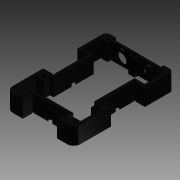
# Autodesk Inventor part: Zwischenebene_Motor2_liegend
Saved by Autodesk Inventor 2015 (Build 190159000, 159)
## iProperties
Created: 2015-03-02
Part Number: Zwischenebene_Motor2_liegend
Material: Generisch
Document SubType Name: Modeling
Designer: TowerSebi
Density: 1 g/cm^3
Appearance: Glatt - schwarz
Author: TowerSebi
Autodesk Inventor part; units mm, degrees
ref_plane "YZ Plane" through (0, 0, 0) normal (1, 0, 0) x (0, 1, 0)
ref_plane "XZ Plane" through (0, 0, 0) normal (0, 1, 0) x (-1, 0, 0)
ref_plane "XY Plane" through (0, 0, 0) normal (0, 0, 1) x (1, 0, 0)
sketch "Skizze1" plane through (0, 0, 0) normal (0, 0, 1) x (1, 0, 0)
  line L0 (0, 0) -> (100, 0)
  line L1 (100, 0) -> (100, 145)
  line L2 (0, 145) -> (0, 0)
  arc A0 (100, 145) -> (0, 145) centre (50, 69.1667) ccw
  dimension "d0" = 145
  dimension "d1" = 100
  constraints: 6 end point, 2 point on circle, 1 centre point, 1 horizontal, 1 parallel, 1 perpendicular
  measures "d0" distance of L2.start L0.start
  measures "d1" distance of L1.end L2.start
extrude "Extrusion1" add sketch "Skizze1" along normal blind 24.5
fillet "Rundung2" radius 10 2 edges at (100, 0, 12.25) (0, 0, 12.25)
fillet "Rundung3" radius 5 2 edges at (100, 145, 12.25) (0, 145, 12.25)
sketch "Skizze3" plane through (0, 0, 0) normal (0, 0, -1) x (-1, 0, 0)
  line L0 (-10, 0) -> (-90, 0) projected
  line L1 (0, 142.2581) -> (0, 10) projected
  circle A0 centre (-90, 10) radius 1.75
  circle A1 centre (-70, 10) radius 1.75
  circle A2 centre (-30, 10) radius 1.75
  circle A3 centre (-10, 10) radius 1.75
  circle A4 centre (-10, 60) radius 1.75
  circle A5 centre (-10, 100) radius 1.75
  circle A6 centre (-10, 140) radius 1.75
  circle A7 centre (-50, 140) radius 1.75
  circle A8 centre (-90, 140) radius 1.75
  circle A9 centre (-90, 100) radius 1.75
  circle A10 centre (-90, 60) radius 1.75
  point P0 (0, 0)
  dimension "d12" = 3.5
  dimension "d13" = 3.5
  dimension "d14" = 3.5
  dimension "d15" = 3.5
  dimension "d16" = 3.5
  dimension "d17" = 3.5
  dimension "d18" = 3.5
  dimension "d19" = 3.5
  dimension "d20" = 3.5
  dimension "d21" = 3.5
  dimension "d22" = 3.5
  dimension "d23" = 140
  dimension "d24" = 140
  dimension "d25" = 140
  dimension "d26" = 100
  dimension "d27" = 100
  dimension "d28" = 60
  dimension "d29" = 60
  dimension "d30" = 10
  dimension "d31" = 10
  dimension "d32" = 10
  dimension "d33" = 10
  dimension "d34" = 90
  dimension "d35" = 70
  dimension "d36" = 30
  dimension "d37" = 10
  dimension "d38" = 90
  dimension "d39" = 10
  dimension "d40" = 90
  dimension "d41" = 10
  dimension "d42" = 90
  dimension "d43" = 50
  dimension "d44" = 10
  constraints: 11 centre point
  measures "d12" diameter of A8
  measures "d13" diameter of A7
  measures "d14" diameter of A6
  measures "d15" diameter of A9
  measures "d16" diameter of A5
  measures "d17" diameter of A10
  measures "d18" diameter of A4
  measures "d19" diameter of A0
  measures "d20" diameter of A1
  measures "d21" diameter of A2
  measures "d22" diameter of A3
  measures "d23" distance from line of L0 A8.centre
  measures "d24" distance from line of L0 A7.centre
  measures "d25" distance from line of L0 A6.centre
  measures "d26" distance from line of L0 A9.centre
  measures "d27" distance from line of L0 A5.centre
  measures "d28" distance from line of L0 A10.centre
  measures "d29" distance from line of L0 A4.centre
  measures "d30" distance from line of L0 A0.centre
  measures "d31" distance from line of A1.centre L0
  measures "d32" distance from line of L0 A2.centre
  measures "d33" distance from line of L0 A3.centre
  measures "d34" distance from line of L1 A0.centre
  measures "d35" distance from line of L1 A1.centre
  measures "d36" distance from line of A2.centre L1
  measures "d37" distance of L1.end A3.centre
  measures "d38" distance from line of L1 A10.centre
  measures "d39" distance from line of L1 A4.centre
  measures "d40" distance from line of L1 A9.centre
  measures "d41" distance from line of L1 A5.centre
  measures "d42" distance from line of A8.centre L1
  measures "d43" distance from line of L1 A7.centre
  measures "d44" distance from line of L1 A6.centre
extrude "Extrusion2" cut sketch "Skizze3" against normal up to next
sketch "Skizze10" plane through (0, 0, 24.5) normal (0, 0, 1) x (1, 0, 0)
  line L0 (0, 142.2581) -> (0, 10) projected
  line L1 (10, 0) -> (90, 0) projected
  line L2 (100, 10) -> (100, 142.2581) projected
  arc A0 (97.6214, 146.5159) -> (2.3786, 146.5159) centre (50, 69.1667) ccw projected
  line L3 (5, 135) -> (5, 110)
  line L4 (5, 110) -> (20.1, 110)
  line L5 (20.1, 110) -> (20.1, 50)
  line L6 (20.1, 50) -> (5, 50)
  line L7 (5, 50) -> (5, 15)
  line L8 (20, 10) -> (20, 20.1)
  line L9 (20, 20.1) -> (80.1, 20.1)
  line L10 (80.1, 20.1) -> (80.1, 10.1)
  line L11 (95.1, 15.1) -> (95.1, 50)
  line L12 (95.1, 50) -> (80, 50)
  line L13 (80, 50) -> (80, 110)
  line L14 (80, 110) -> (95, 110)
  line L15 (95, 110) -> (95, 135)
  line L16 (95, 135) -> (85, 135)
  line L17 (85, 135) -> (85, 140)
  line L18 (85, 140) -> (55, 140)
  line L19 (55, 140) -> (55, 135)
  line L20 (55, 135) -> (45, 135)
  line L21 (45, 135) -> (45, 140)
  line L22 (45, 140) -> (15, 140)
  line L23 (15, 140) -> (15, 135)
  line L24 (15, 135) -> (5, 135)
  line L25 (5, 15) -> (15, 15)
  line L26 (15, 15) -> (15, 10)
  line L27 (15, 10) -> (20, 10)
  line L28 (80.1, 10.1) -> (85.1, 10.1)
  line L29 (85.1, 10.1) -> (85.1, 15.1)
  line L30 (85.1, 15.1) -> (95.1, 15.1)
  line L31 (14.8779, 148) -> (14.8779, 144)
  line L32 (14.8779, 144) -> (85.1221, 144)
  line L33 (85.1221, 144) -> (85.1221, 148)
  line L34 (14.8779, 148) -> (4.8779, 148)
  line L35 (85.1221, 148) -> (95.1221, 148)
  line L36 (0, 105.05) -> (15.1, 105.05)
  line L37 (15.1, 105.05) -> (15.1, 54.95)
  line L38 (15.1, 54.95) -> (0, 54.95)
  line L39 (100, 105.05) -> (84.9, 105.05)
  line L40 (84.9, 105.05) -> (84.9, 54.95)
  line L41 (84.9, 54.95) -> (100, 54.95)
  line L42 (24.95, 0) -> (24.95, 15.1)
  line L43 (24.95, 15.1) -> (75.05, 15.1)
  line L44 (75.05, 15.1) -> (75.05, 0)
  line L45 (15, 50) -> (15, 40)
  line L46 (15, 40) -> (5, 40)
  line L47 (85.1, 50) -> (85.1, 40)
  line L48 (85.1, 40) -> (95.1, 40)
  circle A1 centre (10, 45) radius 1.75
  circle A2 centre (90, 45) radius 1.75
  point P0 (0, 0)
  dimension "d120" = 10
  dimension "d121" = 10
  dimension "d125" = 10.1
  dimension "d128" = 10
  dimension "d129" = 10
  dimension "d130" = 10
  dimension "d131" = 5
  dimension "d132" = 5
  dimension "d133" = 10
  dimension "d134" = 30
  dimension "d135" = 30
  dimension "d137" = 5
  dimension "d138" = 5
  dimension "d139" = 25
  dimension "d140" = 25
  dimension "d141" = 5
  dimension "d142" = 5
  dimension "d143" = 5
  dimension "d144" = 5
  dimension "d145" = 60
  dimension "d146" = 60
  dimension "d149" = 5
  dimension "d150" = 10
  dimension "d152" = 4
  dimension "d154" = 4
  dimension "d155" = 4
  dimension "d158" = 5
  dimension "d159" = 15
  dimension "d160" = 15.1
  dimension "d161" = 15.1
  dimension "d162" = 15.1
  dimension "d163" = 50.1
  dimension "d164" = 15.1
  dimension "d165" = 50.1
  dimension "d166" = 4.95
  dimension "d167" = 4.95
  dimension "d168" = 15.1
  dimension "d170" = 50
  dimension "d171" = 50.1
  dimension "d172" = 4.95
  dimension "d173" = 5.05
  dimension "d177" = 10
  dimension "d178" = 10
  dimension "d179" = 10
  dimension "d180" = 10
  dimension "d181" = 3.5
  dimension "d182" = 3.5
  dimension "d183" = 45
  dimension "d184" = 45
  dimension "d185" = 10
  dimension "d186" = 10
  dimension "d191" = 10
  dimension "d192" = 10
  constraints: 92 end point, 28 parallel, 13 perpendicular, 10 point on line, 2 centre point, 2 collinear, 2 point on circle
  measures "d120" distance of L23.end L3.start
  measures "d121" distance of L15.end L16.end
  measures "d125" distance of L8.start L8.end
  measures "d128" distance of L9.end L10.end
  measures "d129" distance of L29.end L11.start
  measures "d130" distance of L7.end L25.end
  measures "d131" distance of L25.end L26.end
  measures "d132" distance of L28.end L29.end
  measures "d133" distance of L19.end L20.end
  measures "d134" distance of L21.end L22.end
  measures "d135" distance of L17.end L18.end
  measures "d137" distance of L26.end L8.start
  measures "d138" distance of L10.end L28.end
  measures "d139" distance of L3.start L3.end
  measures "d140" distance of L14.end L15.end
  measures "d141" distance of L22.end L23.end
  measures "d142" distance of L18.end L19.end
  measures "d143" distance of L20.end L21.end
  measures "d144" distance of L16.end L17.end
  measures "d145" distance of L4.end L5.end
  measures "d146" distance of L12.end L13.end
  measures "d149" distance between parallel lines of L0 L7
  measures "d150" distance between parallel lines of L1 L27
  measures "d152" distance between parallel lines of L32 L22
  measures "d154" distance between parallel lines of L32 L34
  measures "d155" distance between parallel lines of L32 L35
  measures "d158" distance between parallel lines of L0 L3
  measures "d159" distance of L13.end L14.end
  measures "d160" distance of L11.end L12.end
  measures "d161" distance of L5.end L6.end
  measures "d162" distance of L36.start L36.end
  measures "d163" distance of L36.end L37.end
  measures "d164" distance of L39.start L39.end
  measures "d165" distance of L39.end L40.end
  measures "d166" distance between parallel lines of L39 L14
  measures "d167" distance between parallel lines of L4 L36
  measures "d168" distance of L42.start L42.end
  measures "d170" distance between parallel lines of L1 L6
  measures "d171" distance of L42.end L43.end
  measures "d172" distance between parallel lines of L42 L8
  measures "d173" distance between parallel lines of L10 L44
  measures "d177" distance of L45.start L45.end
  measures "d178" distance of L45.end L46.end
  measures "d179" distance of L47.end L48.end
  measures "d180" distance of L47.start L47.end
  measures "d181" diameter of A1
  measures "d182" diameter of A2
  measures "d183" distance from line of L1 A1.centre
  measures "d184" distance from line of L1 A2.centre
  measures "d185" distance from line of A2.centre L2
  measures "d186" distance from line of L0 A1.centre
  measures "d191" distance of L31.start L34.end
  measures "d192" distance of L33.end L35.end
extrude "Extrusion11" cut sketch "Skizze10" against normal up to next contours L36 L37 L38 L0 | L42 L43 L44 L1 | L41 L40 L39 L2 | L35 L33 L32 L31 L34 A0 | L24 L23 L22 L21 L20 L19 L18 L17 L16 L15 L14 L13 L12 L47 L48 L11 L30 L29 L28 L10 L9 L8 L27 L26 L25 L7 L46 L45 L6 L5 L4 L3 | A1 | A2
fillet "Rundung8" radius 1 31 edges at (15, 40, 12.25) (20.1, 50, 12.25) (5, 40, 12.25) (20.1, 110, 12.25) (5, 135, 12.25) (5, 110, 12.25) (15, 135, 12.25) (15, 140, 12.25) (5, 15, 12.25) (15, 15, 12.25) (15, 10, 12.25) (20, 10, 12.25) (20, 20.1, 12.25) (80.1, 20.1, 12.25) (80.1, 10.1, 12.25) (85.1, 10.1, 12.25) (85.1, 15.1, 12.25) (95.1, 15.1, 12.25) (95.1, 40, 12.25) (85.1, 40, 12.25) (85.1, 50, 12.25) (80, 50, 12.25) (80, 110, 12.25) (95, 110, 12.25) (95, 135, 12.25) (85, 135, 12.25) (85, 140, 12.25) (55, 140, 12.25) (55, 135, 12.25) (45, 135, 12.25) (45, 140, 12.25)
fillet "Rundung9" radius 1 4 edges at (14.8779, 148, 12.25) (85.1221, 148, 12.25) (85.1221, 144, 12.25) (14.8779, 144, 12.25)
sketch "Skizze11" plane through (15.8779, 144, 24.5) normal (0, 1, 0) x (1, 0, 0)
  line L0 (0, 0) -> (0, 24.5) projected
  line L1 (68.2441, 0) -> (0, 0) projected
  line L2 (68.2441, 24.5) -> (68.2441, 0) projected
  line L3 (0, 24.5) -> (68.2441, 24.5) projected
  circle A0 centre (14.25, 15.5) radius 7.75
  circle A1 centre (3, 15.5) radius 1.65
  circle A2 centre (25.5, 15.5) radius 1.65
  line L4 (9.75, 6.25) -> (18.75, 6.25)
  line L5 (18.75, 6.25) -> (18.75, 1.75)
  line L6 (18.75, 1.75) -> (9.75, 1.75)
  line L7 (9.75, 1.75) -> (9.75, 6.25)
  circle A3 centre (4.75, 4) radius 1.1
  circle A4 centre (47.2441, 15.5) radius 3.5
  circle A5 centre (60.2441, 15.5) radius 2.5
  circle A6 centre (44.2441, 5) radius 1.1514
  line L8 (49.2441, 7.25) -> (58.2441, 7.25)
  line L9 (58.2441, 7.25) -> (58.2441, 2.75)
  line L10 (58.2441, 2.75) -> (49.2441, 2.75)
  line L11 (49.2441, 2.75) -> (49.2441, 7.25)
  circle A7 centre (23.75, 4) radius 1.1
  circle A8 centre (63.2441, 5) radius 1.1514
  point P0 (-15.8779, 24.5)
  dimension "d193" = 15.5
  dimension "d194" = 3.3
  dimension "d195" = 3.3
  dimension "d196" = 22.5
  dimension "d197" = 11.25
  dimension "d200" = 2.2
  dimension "d202" = 7
  dimension "d203" = 5
  dimension "d212" = 9
  dimension "d213" = 3
  dimension "d215" = 4.5
  dimension "d216" = 5
  dimension "d217" = 2.2
  dimension "d219" = 5
  dimension "d220" = 4.5
  dimension "d221" = 9
  dimension "d222" = 2.75
  dimension "d223" = 1.75
  dimension "d224" = 2.25
  dimension "d225" = 2.25
  dimension "d226" = 2.25
  dimension "d227" = 2.25
  dimension "d228" = 5
  dimension "d229" = 5
  dimension "d230" = 5
  dimension "d231" = 8
  dimension "d232" = 21
  dimension "d235" = 9
  dimension "d236" = 9
  dimension "d237" = 9
  dimension "d238" = 9
  dimension "d377" = 4.5
  dimension "d378" = 4.5
  constraints: 16 end point, 9 centre point, 4 parallel, 2 horizontal, 2 perpendicular
  measures "d193" diameter of A0
  measures "d194" diameter of A1
  measures "d195" diameter of A2
  measures "d196" distance of A1.centre A2.centre
  measures "d197" distance of A0.centre A1.centre
  measures "d200" diameter of A3
  measures "d202" diameter of A4
  measures "d203" diameter of A5
  measures "d212" distance from line of L3 A1.centre
  measures "d213" distance from line of L0 A1.centre
  measures "d215" distance of L6.end L4.start
  measures "d216" distance from line of L7 A3.centre
  measures "d217" diameter of A7
  measures "d219" distance from line of L5 A7.centre
  measures "d220" distance of L8.end L10.start
  measures "d221" distance of L10.start L11.start
  measures "d222" distance between parallel lines of L1 L10
  measures "d223" distance between parallel lines of L1 L6
  measures "d224" distance from line of L10 A8.centre
  measures "d225" distance from line of L10 A6.centre
  measures "d226" distance from line of L6 A7.centre
  measures "d227" distance from line of L6 A3.centre
  measures "d228" distance from line of A6.centre L11
  measures "d229" distance from line of L9 A8.centre
  measures "d230" distance from line of L2 A8.centre
  measures "d231" distance from line of L2 A5.centre
  measures "d232" distance from line of L2 A4.centre
  measures "d235" distance from line of L3 A0.centre
  measures "d236" distance from line of L3 A2.centre
  measures "d237" distance from line of L3 A4.centre
  measures "d238" distance from line of L3 A5.centre
  measures "d377" distance from line of A0.centre L5
  measures "d378" distance from line of A0.centre L7
extrude "Extrusion12" cut sketch "Skizze11" against normal blind 10 contours A0 | A1 | A2 | L4 L5 L6 L7 | A3 | A4 | A5 | A6 | L8 L9 L10 L11 | A7 | A8
hole "Bohrung2" at (10, 45, 24.5) direction (0, 0, -1) diameter 3.4 end through all counterbore diameter 6.5 counterbore depth 4 clearance for "Inbusschraube DIN EN ISO 4762" size "M3" standard "DIN"
hole "Bohrung3" at (90, 45, 24.5) direction (0, 0, -1) diameter 3.4 end through all counterbore diameter 6.5 counterbore depth 4 clearance for "Inbusschraube DIN EN ISO 4762" size "M3" standard "DIN"
hole "Bohrung4" at (50, 140, 24.5) direction (0, 0, -1) diameter 3.4 end through all counterbore diameter 6.5 counterbore depth 4 clearance for "Inbusschraube DIN EN ISO 4762" size "M3" standard "DIN"
sketch "Skizze12" plane through (0, 0, 0) normal (0, 0, -1) x (-1, 0, 0)
  line L0 (-84.9, 105.05) -> (-84.9, 54.95) projected
  line L1 (-84.9, 54.95) -> (-100, 54.95) projected
  line L2 (-75.05, 15.1) -> (-24.95, 15.1) projected
  line L3 (-24.95, 15.1) -> (-24.95, 0) projected
  line L4 (0, 54.95) -> (-15.1, 54.95) projected
  line L5 (-15.1, 54.95) -> (-15.1, 105.05) projected
  line L6 (-80.6, 84.15) -> (-84.4, 84.15)
  line L7 (-84.4, 84.15) -> (-84.4, 76.15)
  line L8 (-84.4, 76.15) -> (-80.6, 76.15)
  line L9 (-80.6, 76.15) -> (-80.6, 84.15)
  line L10 (-19.4, 84.15) -> (-15.6, 84.15)
  line L11 (-15.6, 84.15) -> (-15.6, 76.15)
  line L12 (-15.6, 76.15) -> (-19.4, 76.15)
  line L13 (-19.4, 76.15) -> (-19.4, 84.15)
  line L14 (-53.95, 19.4) -> (-45.95, 19.4)
  line L15 (-45.95, 19.4) -> (-45.95, 15.6)
  line L16 (-45.95, 15.6) -> (-53.95, 15.6)
  line L17 (-53.95, 15.6) -> (-53.95, 19.4)
  point P0 (0, 0)
  dimension "d266" = 8
  dimension "d267" = 8
  dimension "d268" = 8
  dimension "d269" = 3.8
  dimension "d270" = 3.8
  dimension "d271" = 3.8
  dimension "d272" = 0.5
  dimension "d273" = 0.5
  dimension "d274" = 0.5
  dimension "d275" = 21.2
  dimension "d276" = 21.2
  dimension "d277" = 21
  constraints: 24 end point, 6 parallel, 3 horizontal, 3 perpendicular
  measures "d266" distance of L6.end L7.end
  measures "d267" distance of L12.end L10.start
  measures "d268" distance of L15.end L16.end
  measures "d269" distance of L6.start L6.end
  measures "d270" distance of L11.end L12.end
  measures "d271" distance of L16.end L14.start
  measures "d272" distance between parallel lines of L0 L7
  measures "d273" distance between parallel lines of L5 L11
  measures "d274" distance between parallel lines of L2 L16
  measures "d275" distance between parallel lines of L1 L8
  measures "d276" distance between parallel lines of L4 L12
  measures "d277" distance between parallel lines of L3 L15
extrude "Extrusion13" cut sketch "Skizze12" against normal blind 6
sketch "Skizze17" plane through (0, 0, 0) normal (0, 0, -1) x (-1, 0, 0)
  line L0 (-100, 105.05) -> (-100, 142.2581) projected
  line L1 (-100, 105.05) -> (-84.9, 105.05) projected
  line L2 (-84.9, 105.05) -> (-84.9, 54.95) projected
  line L3 (-84.9, 54.95) -> (-100, 54.95) projected
  line L4 (-100, 10) -> (-100, 54.95) projected
  line L5 (-75.05, 0) -> (-90, 0) projected
  line L6 (-75.05, 0) -> (-75.05, 15.1) projected
  line L7 (-75.05, 15.1) -> (-24.95, 15.1) projected
  line L8 (-24.95, 15.1) -> (-24.95, 0) projected
  line L9 (-10, 0) -> (-24.95, 0) projected
  line L10 (0, 54.95) -> (0, 10) projected
  line L11 (0, 54.95) -> (-15.1, 54.95) projected
  line L12 (-15.1, 54.95) -> (-15.1, 105.05) projected
  line L13 (-15.1, 105.05) -> (0, 105.05) projected
  line L14 (0, 142.2581) -> (0, 105.05) projected
  line L15 (-85.1221, 145) -> (-85.1221, 147) projected
  line L16 (-100, 105.1) -> (-84.8, 105.1)
  line L17 (-84.8, 105.1) -> (-84.8, 54.9)
  line L18 (-84.8, 54.9) -> (-100, 54.9)
  line L19 (0, 105.1) -> (-15.2, 105.1)
  line L20 (-15.2, 105.1) -> (-15.2, 54.9)
  line L21 (-15.2, 54.9) -> (0, 54.9)
  line L22 (-75.1, 0) -> (-75.1, 15.2)
  line L23 (-75.1, 15.2) -> (-24.9, 15.2)
  line L24 (-24.9, 15.2) -> (-24.9, 0)
  point P0 (0, 0)
  dimension "d342" = 0.05
  dimension "d343" = 0.05
  dimension "d344" = 0.1
  dimension "d345" = 0.1
  dimension "d347" = 0.05
  dimension "d348" = 0.05
  dimension "d349" = 0.05
  dimension "d350" = 0.05
  dimension "d351" = 0.1
  constraints: 18 end point, 7 perpendicular, 6 point on line, 2 parallel
  measures "d342" distance between parallel lines of L6 L22
  measures "d343" distance between parallel lines of L8 L24
  measures "d344" distance between parallel lines of L7 L23
  measures "d345" distance between parallel lines of L17 L2
  measures "d347" distance between parallel lines of L11 L21
  measures "d348" distance between parallel lines of L3 L18
  measures "d349" distance between parallel lines of L16 L1
  measures "d350" distance between parallel lines of L13 L19
  measures "d351" distance between parallel lines of L12 L20
extrude "Extrusion20" cut sketch "Skizze17" against normal blind 30
sketch "Skizze13" plane through (0, 0, 0) normal (0, 0, -1) x (-1, 0, 0)
  line L0 (-19.4, 76.15) -> (-19.4, 84.15) projected
  line L1 (-19.4, 84.15) -> (-15.6, 84.15) projected
  line L2 (-15.6, 84.15) -> (-15.6, 76.15) projected
  line L3 (-15.6, 76.15) -> (-19.4, 76.15) projected
  line L4 (-84.4, 76.15) -> (-84.4, 84.15) projected
  line L5 (-84.4, 84.15) -> (-80.6, 84.15) projected
  line L6 (-80.6, 84.15) -> (-80.6, 76.15) projected
  line L7 (-80.6, 76.15) -> (-84.4, 76.15) projected
  line L8 (-53.95, 15.6) -> (-53.95, 19.4) projected
  line L9 (-53.95, 19.4) -> (-45.95, 19.4) projected
  line L10 (-45.95, 19.4) -> (-45.95, 15.6) projected
  line L11 (-45.95, 15.6) -> (-53.95, 15.6) projected
  line L12 (-20.1, 109) -> (-20.1, 51) projected
  line L13 (-21, 20.1) -> (-79.1, 20.1) projected
  line L14 (-80, 51) -> (-80, 109) projected
  line L15 (-84.9, 105.05) -> (-84.9, 54.95) projected
  line L16 (-75.05, 15.1) -> (-24.95, 15.1) projected
  line L17 (-15.1, 54.95) -> (-15.1, 105.05) projected
  line L18 (-15.6, 83.34) -> (-15.1, 83.34)
  line L19 (-15.1, 83.34) -> (-15.1, 82.34)
  line L20 (-15.1, 82.34) -> (-15.6, 82.34)
  line L21 (-15.6, 82.34) -> (-15.6, 83.34)
  line L22 (-15.6, 80.5) -> (-15.1, 80.5)
  line L23 (-15.1, 80.5) -> (-15.1, 79.5)
  line L24 (-15.1, 79.5) -> (-15.6, 79.5)
  line L25 (-15.6, 79.5) -> (-15.6, 80.5)
  line L26 (-15.6, 76.96) -> (-15.1, 76.96)
  line L27 (-15.1, 76.96) -> (-15.1, 77.96)
  line L28 (-15.1, 77.96) -> (-15.6, 77.96)
  line L29 (-15.6, 77.96) -> (-15.6, 76.96)
  line L30 (-19.4, 83.34) -> (-20.1, 83.34)
  line L31 (-20.1, 83.34) -> (-20.1, 82.34)
  line L32 (-20.1, 82.34) -> (-19.4, 82.34)
  line L33 (-19.4, 82.34) -> (-19.4, 83.34)
  line L34 (-19.4, 80.8) -> (-20.1, 80.8)
  line L35 (-20.1, 80.8) -> (-20.1, 79.8)
  line L36 (-20.1, 79.8) -> (-19.4, 79.8)
  line L37 (-19.4, 79.8) -> (-19.4, 80.8)
  line L38 (-19.4, 77.96) -> (-20.1, 77.96)
  line L39 (-20.1, 77.96) -> (-20.1, 76.96)
  line L40 (-20.1, 76.96) -> (-19.4, 76.96)
  line L41 (-19.4, 76.96) -> (-19.4, 77.96)
  line L42 (-84.9, 83.34) -> (-84.4, 83.34)
  line L43 (-84.4, 83.34) -> (-84.4, 82.34)
  line L44 (-84.4, 82.34) -> (-84.9, 82.34)
  line L45 (-84.9, 82.34) -> (-84.9, 83.34)
  line L46 (-84.9, 80.5) -> (-84.4, 80.5)
  line L47 (-84.4, 80.5) -> (-84.4, 79.5)
  line L48 (-84.4, 79.5) -> (-84.9, 79.5)
  line L49 (-84.9, 79.5) -> (-84.9, 80.5)
  line L50 (-84.9, 77.96) -> (-84.4, 77.96)
  line L51 (-84.4, 77.96) -> (-84.4, 76.96)
  line L52 (-84.4, 76.96) -> (-84.9, 76.96)
  line L53 (-84.9, 76.96) -> (-84.9, 77.96)
  line L54 (-80.6, 76.96) -> (-80, 76.96)
  line L55 (-80, 76.96) -> (-80, 77.96)
  line L56 (-80, 77.96) -> (-80.6, 77.96)
  line L57 (-80.6, 77.96) -> (-80.6, 76.96)
  line L58 (-80.6, 79.5) -> (-80, 79.5)
  line L59 (-80, 79.5) -> (-80, 80.5)
  line L60 (-80, 80.5) -> (-80.6, 80.5)
  line L61 (-80.6, 80.5) -> (-80.6, 79.5)
  line L62 (-80.6, 82.34) -> (-80, 82.34)
  line L63 (-80, 82.34) -> (-80, 83.34)
  line L64 (-80, 83.34) -> (-80.6, 83.34)
  line L65 (-80.6, 83.34) -> (-80.6, 82.34)
  line L66 (-53.14, 20.1) -> (-52.14, 20.1)
  line L67 (-52.14, 20.1) -> (-52.14, 19.4)
  line L68 (-52.14, 19.4) -> (-53.14, 19.4)
  line L69 (-53.14, 19.4) -> (-53.14, 20.1)
  line L70 (-50.6, 20.1) -> (-49.6, 20.1)
  line L71 (-49.6, 20.1) -> (-49.6, 19.4)
  line L72 (-49.6, 19.4) -> (-50.6, 19.4)
  line L73 (-50.6, 19.4) -> (-50.6, 20.1)
  line L74 (-47.76, 20.1) -> (-46.76, 20.1)
  line L75 (-46.76, 20.1) -> (-46.76, 19.4)
  line L76 (-46.76, 19.4) -> (-47.76, 19.4)
  line L77 (-47.76, 19.4) -> (-47.76, 20.1)
  line L78 (-46.76, 15.6) -> (-47.76, 15.6)
  line L79 (-47.76, 15.6) -> (-47.76, 15.1)
  line L80 (-47.76, 15.1) -> (-46.76, 15.1)
  line L81 (-46.76, 15.1) -> (-46.76, 15.6)
  line L82 (-52.14, 15.6) -> (-53.14, 15.6)
  line L83 (-53.14, 15.6) -> (-53.14, 15.1)
  line L84 (-53.14, 15.1) -> (-52.14, 15.1)
  line L85 (-52.14, 15.1) -> (-52.14, 15.6)
  line L86 (-50.6, 15.6) -> (-49.6, 15.6)
  line L87 (-49.6, 15.6) -> (-49.6, 15.1)
  line L88 (-49.6, 15.1) -> (-50.6, 15.1)
  line L89 (-50.6, 15.1) -> (-50.6, 15.6)
  point P0 (0, 0)
  dimension "d280" = 1
  dimension "d281" = 1
  dimension "d282" = 1
  dimension "d283" = 1
  dimension "d284" = 1
  dimension "d285" = 1
  dimension "d286" = 0.81
  dimension "d287" = 0.81
  dimension "d288" = 0.81
  dimension "d289" = 0.81
  dimension "d290" = 1.54
  dimension "d291" = 1.84
  dimension "d292" = 1.54
  dimension "d293" = 1.84
  dimension "d294" = 0.81
  dimension "d295" = 0.81
  dimension "d296" = 0.81
  dimension "d297" = 0.81
  dimension "d298" = 1.54
  dimension "d299" = 1.54
  dimension "d300" = 1
  dimension "d301" = 1
  dimension "d302" = 1
  dimension "d303" = 1
  dimension "d304" = 1
  dimension "d305" = 1
  dimension "d306" = 1.84
  dimension "d307" = 1.84
  dimension "d308" = 0.81
  dimension "d309" = 0.81
  dimension "d310" = 0.81
  dimension "d311" = 0.81
  dimension "d312" = 1
  dimension "d313" = 1
  dimension "d314" = 1
  dimension "d315" = 1
  dimension "d317" = 1
  dimension "d318" = 1.54
  dimension "d320" = 1
  dimension "d321" = 1.54
  dimension "d322" = 1.84
  dimension "d323" = 1.84
  constraints: 144 end point, 36 parallel, 36 point on line, 18 horizontal, 18 perpendicular
  measures "d280" distance between parallel lines of L20 L18
  measures "d281" distance between parallel lines of L24 L22
  measures "d282" distance between parallel lines of L26 L28
  measures "d283" distance between parallel lines of L32 L30
  measures "d284" distance between parallel lines of L36 L34
  measures "d285" distance between parallel lines of L40 L38
  measures "d286" distance between parallel lines of L18 L1
  measures "d287" distance between parallel lines of L3 L26
  measures "d288" distance between parallel lines of L1 L30
  measures "d289" distance between parallel lines of L3 L40
  measures "d290" distance between parallel lines of L24 L28
  measures "d291" distance between parallel lines of L20 L22
  measures "d292" distance between parallel lines of L34 L32
  measures "d293" distance between parallel lines of L36 L38
  measures "d294" distance between parallel lines of L5 L42
  measures "d295" distance between parallel lines of L5 L64
  measures "d296" distance between parallel lines of L7 L54
  measures "d297" distance between parallel lines of L7 L52
  measures "d298" distance between parallel lines of L48 L50
  measures "d299" distance between parallel lines of L58 L56
  measures "d300" distance between parallel lines of L52 L50
  measures "d301" distance between parallel lines of L54 L56
  measures "d302" distance between parallel lines of L58 L60
  measures "d303" distance between parallel lines of L48 L46
  measures "d304" distance between parallel lines of L42 L44
  measures "d305" distance between parallel lines of L62 L64
  measures "d306" distance between parallel lines of L60 L62
  measures "d307" distance between parallel lines of L46 L44
  measures "d308" distance between parallel lines of L69 L8
  measures "d309" distance between parallel lines of L10 L75
  measures "d310" distance between parallel lines of L10 L81
  measures "d311" distance between parallel lines of L8 L83
  measures "d312" distance between parallel lines of L69 L67
  measures "d313" distance between parallel lines of L75 L77
  measures "d314" distance between parallel lines of L81 L79
  measures "d315" distance between parallel lines of L83 L85
  measures "d317" distance between parallel lines of L71 L73
  measures "d318" distance between parallel lines of L73 L67
  measures "d320" distance between parallel lines of L87 L89
  measures "d321" distance between parallel lines of L85 L89
  measures "d322" distance between parallel lines of L79 L87
  measures "d323" distance between parallel lines of L77 L71
extrude "Extrusion14" [suppressed]
sketch "Skizze14" plane through (0, 0, 0) normal (0, 0, -1) x (-1, 0, 0)
  line L0 (-53.04, 15.1) -> (-53.04, 15.9) projected
  line L1 (-45.95, 15.6) -> (-53.95, 15.6) projected
  line L2 (-84.9, 105.05) -> (-84.9, 54.95) projected
  line L3 (-75.05, 15.1) -> (-24.95, 15.1) projected
  line L4 (-53.04, 15.9) -> (-46.15, 15.9)
  line L5 (-46.15, 15.9) -> (-46.15, 15.0908)
  line L6 (-46.15, 15.0908) -> (-53.04, 15.0908)
  line L7 (-53.04, 15.0908) -> (-53.04, 15.9)
  line L8 (-53.95, 15.6) -> (-53.95, 15.1)
  line L9 (-84.4, 76.15) -> (-84.9, 76.15)
  line L10 (-84.9, 76.15) -> (-84.3999, 76.15)
  line L11 (-84.3999, 76.15) -> (-84.3999, 83.85)
  line L12 (-84.3999, 83.85) -> (-84.9, 83.85)
  line L13 (-84.9, 83.85) -> (-84.9, 76.15)
  line L14 (-15.9001, 76.15) -> (-15.0942, 76.15)
  line L15 (-15.0942, 76.15) -> (-15.0942, 83.85)
  line L16 (-15.0942, 83.85) -> (-15.9001, 83.85)
  line L17 (-15.9001, 83.85) -> (-15.9001, 76.15)
  point P0 (-84.9, 76.96)
  point P1 (0, 0)
  constraints: 28 end point, 6 parallel, 5 perpendicular, 3 horizontal, 2 point on line, 1 other
extrude "Extrusion15" [suppressed]
sketch "Skizze15" plane through (0, 0, 0) normal (0, 0, -1) x (-1, 0, 0)
  line L0 (-15.6, 76.15) -> (-19.4, 76.15) projected
  line L1 (-80.6, 76.15) -> (-84.4, 76.15) projected
  line L2 (-20.1, 109) -> (-20.1, 51) projected
  line L3 (-80, 51) -> (-80, 109) projected
  line L4 (-84.9, 105.05) -> (-84.9, 54.95) projected
  line L5 (-15.1, 54.95) -> (-15.1, 105.05) projected
  line L6 (-84.9, 83.05) -> (-80, 83.05)
  line L7 (-80, 83.05) -> (-80, 76.95)
  line L8 (-80, 76.95) -> (-84.9, 76.95)
  line L9 (-84.9, 76.95) -> (-84.9, 83.05)
  line L10 (-20.1, 83.05) -> (-15.1, 83.05)
  line L11 (-15.1, 83.05) -> (-15.1, 76.95)
  line L12 (-15.1, 76.95) -> (-20.1, 76.95)
  line L13 (-20.1, 76.95) -> (-20.1, 83.05)
  point P0 (0, 0)
  dimension "d331" = 0.8
  dimension "d333" = 0.8
  dimension "d340" = 6.1
  dimension "d341" = 6.1
  constraints: 16 end point, 4 parallel, 4 point on line, 2 horizontal, 2 perpendicular
  measures "d331" distance between parallel lines of L12 L0
  measures "d333" distance between parallel lines of L8 L1
  measures "d340" distance between parallel lines of L12 L10
  measures "d341" distance between parallel lines of L8 L6
extrude "Extrusion16" cut sketch "Skizze15" against normal blind 4
sketch "Skizze16" plane through (0, 0, 0) normal (0, 0, -1) x (-1, 0, 0)
  line L0 (-21, 20.1) -> (-79.1, 20.1) projected
  line L1 (-75.05, 15.1) -> (-24.95, 15.1) projected
  line L2 (-53.95, 15.6) -> (-53.95, 19.4) projected
  line L3 (-45.95, 19.4) -> (-45.95, 15.6) projected
  line L4 (-53.15, 20.1) -> (-46.75, 20.1)
  line L5 (-46.75, 20.1) -> (-46.75, 15.1)
  line L6 (-46.75, 15.1) -> (-53.15, 15.1)
  line L7 (-53.15, 15.1) -> (-53.15, 20.1)
  point P0 (0, 0)
  dimension "d336" = 0.8
  dimension "d337" = 0.8
  constraints: 8 end point, 2 parallel, 2 point on line, 1 horizontal, 1 perpendicular
  measures "d336" distance between parallel lines of L7 L2
  measures "d337" distance between parallel lines of L5 L3
extrude "Extrusion17" cut sketch "Skizze16" against normal blind 4
sketch "Skizze18" plane through (0, 0, 0) normal (0, 0, -1) x (-1, 0, 0)
  circle A0 centre (-84.8, 105.1) radius 1
  circle A1 centre (-15.2, 105.1) radius 1
  circle A2 centre (-15.2, 54.9002) radius 1
  circle A3 centre (-84.8, 54.9) radius 1
  circle A4 centre (-75.1, 15.2) radius 1
  circle A5 centre (-24.9, 15.2) radius 1
  point P0 (0, 0)
  dimension "d358" = 2
  dimension "d359" = 2
  dimension "d360" = 2
  dimension "d361" = 2
  dimension "d362" = 2
  dimension "d363" = 2
  constraints: 6 centre point, 2 coincident
  measures "d358" diameter of A4
  measures "d359" diameter of A5
  measures "d360" diameter of A2
  measures "d361" diameter of A1
  measures "d362" diameter of A0
  measures "d363" diameter of A3
extrude "Extrusion21" cut sketch "Skizze18" against normal blind 30
sketch "Skizze19" plane through (0, 0, 0) normal (0, 0, -1) x (-1, 0, 0)
  line L0 (-84.4, 84.15) -> (-80.6, 84.15) projected
  line L1 (-19.4, 84.15) -> (-15.6, 84.15) projected
  line L2 (-84.1, 84.45) -> (-80.6, 84.45)
  line L3 (-80.6, 84.45) -> (-80.6, 75.85)
  line L4 (-80.6, 75.85) -> (-84.1, 75.85)
  line L5 (-84.1, 75.85) -> (-84.1, 84.45)
  line L6 (-19.3, 84.45) -> (-16, 84.45)
  line L7 (-16, 84.45) -> (-16, 75.85)
  line L8 (-16, 75.85) -> (-19.3, 75.85)
  line L9 (-19.3, 75.85) -> (-19.3, 84.45)
  line L10 (-80.6, 76.15) -> (-84.4, 76.15) projected
  line L11 (-15.6, 76.15) -> (-19.4, 76.15) projected
  line L12 (-80.6, 84.15) -> (-80.6, 83.05) projected
  point P0 (0, 0)
  dimension "d366" = 0.3
  dimension "d367" = 0.3
  dimension "d368" = 0.3
  dimension "d369" = 0.3
  dimension "d372" = 0
  constraints: 16 end point, 4 parallel, 2 horizontal, 2 perpendicular
  measures "d366" distance between parallel lines of L2 L0
  measures "d367" distance between parallel lines of L1 L6
  measures "d368" distance between parallel lines of L10 L4
  measures "d369" distance between parallel lines of L11 L8
  measures "d372" distance between parallel lines of L3 L12
extrude "Extrusion22" cut sketch "Skizze19" against normal blind 6
